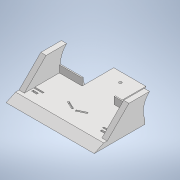
# Autodesk Inventor part: dół
Saved by Autodesk Inventor 2022 (Build 260153000, 153)
## iProperties
Created: 2022-12-08
Part Number: dół
Material: Generic
Document SubType Name: Modeling
Designer: Kamil
Density: 1 g/cm^3
Appearance: Default
Author: Kamil
Autodesk Inventor part; units mm, degrees
ref_plane "YZ Plane" through (0, 0, 0) normal (1, 0, 0) x (0, 1, 0)
ref_plane "XZ Plane" through (0, 0, 0) normal (0, 1, 0) x (-1, 0, 0)
ref_plane "XY Plane" through (0, 0, 0) normal (0, 0, 1) x (1, 0, 0)
sketch "Sketch1" plane through (0, 0, 0) normal (0, 1, 0) x (-1, 0, 0)
  line L0 (-49.6221, -50.9693) -> (50.3779, -50.9693)
  line L1 (50.3779, -50.9693) -> (50.3779, 49.0307)
  line L2 (50.3779, 49.0307) -> (-49.6221, 49.0307)
  line L3 (-49.6221, 49.0307) -> (-49.6221, -50.9693)
  line L4 (-17.8721, -0.5117) -> (18.6279, -0.5117)
  line L5 (18.6279, -0.5117) -> (18.6279, -50.9693)
  line L6 (18.6279, -50.9693) -> (-17.8721, -50.9693)
  line L7 (-17.8721, -50.9693) -> (-17.8721, -0.5117)
  line L8 (-49.6221, -18.7693) -> (50.3779, -18.7693)
  line L9 (50.3779, -18.7693) -> (50.3779, -50.9693)
  line L10 (50.3779, -50.9693) -> (-49.6221, -50.9693)
  line L11 (-49.6221, -50.9693) -> (-49.6221, -18.7693)
  line L12 (-49.6221, -18.7693) -> (50.3779, -18.7693)
  line L13 (50.3779, -18.7693) -> (50.3779, -14.7693)
  line L14 (50.3779, -14.7693) -> (-49.6221, -14.7693)
  line L15 (-49.6221, -14.7693) -> (-49.6221, -18.7693)
  line L16 (-49.6221, -34.8693) -> (50.3779, -34.8693)
  line L17 (-49.6221, -50.9693) -> (50.3779, -50.9693)
  line L18 (50.3779, -50.9693) -> (50.3779, -46.9693)
  line L19 (50.3779, -46.9693) -> (-49.6221, -46.9693)
  line L20 (-49.6221, -46.9693) -> (-49.6221, -50.9693)
  point P0 (0, 0)
  point P1 (0.3779, -50.9693)
  point P2 (0.3779, -50.9693)
  point P3 (0.3779, -50.9693)
  point P4 (-49.6221, -14.7693)
  point P5 (-17.8721, -14.7693)
  point P6 (-17.8721, -46.9693)
  point P7 (18.6279, -46.9693)
  point P8 (18.6279, -14.7693)
  dimension "d0" = 100
  dimension "d1" = 100
  dimension "d2" = 36.5
  dimension "d3" = 100
  dimension "d4" = 32.2
  dimension "d5" = 4
  dimension "d6" = 4
  constraints: 42 end point, 10 parallel, 5 horizontal, 5 midpoint, 5 perpendicular, 2 point on line
  measures "d0" distance of L2.end L1.end
  measures "d1" distance of L1.end L0.end
  measures "d2" distance of L5.end L6.end
  measures "d3" distance of L9.end L10.end
  measures "d4" distance of L8.end L9.end
  measures "d5" distance of L13.end L12.end
  measures "d6" distance of L18.end L17.end
extrude "Extrusion1" add sketch "Sketch1" along normal blind 4 contours L7 L16 L5 L19 | L7 L8 L5 L16 | L7 L14 L5 L8 | L3 L2 L1 L14 L5 L4 L7 | L7 L4 L5 L14
sketch "Sketch2" plane through (17.8721, 0, -14.7693) normal (1, 0, 0) x (0, 0, -1)
  line L0 (0, 0) -> (32.2, 0) projected
  line L1 (32.2, 0) -> (32.2, 4) projected
  line L2 (0, 4) -> (32.2, 4) projected
  line L3 (0, 0) -> (0, 4) projected
  circle A0 centre (20.1, 13.6) radius 16.1 projected
  line L4 (32.2, 0) -> (32.2, 4) projected
  circle A1 centre (20.1, 13.6) radius 15.4457
  point P0 (-14.7693, 0)
  point P1 (27.4219, 0)
  constraints: 1 coincident, 3 other
extrude "Extrusion2" cut sketch "Sketch2" against normal through all contours A0 L1 L0 | L0 A1 L1 A0
sketch "Sketch3" plane through (0, 0, 0) normal (0, -1, 0) x (1, 0, 0)
  line L0 (-18.6279, -46.9693) -> (-18.6279, -42.1911) projected
  line L1 (17.8721, -46.9693) -> (-18.6279, -46.9693) projected
  line L2 (17.8721, -42.1911) -> (17.8721, -46.9693) projected
  line L3 (-18.6279, -42.1911) -> (17.8721, -42.1911) projected
  line L4 (-18.6279, -42.1911) -> (17.8721, -42.1911) projected
  line L5 (17.8721, -14.7693) -> (17.8721, -42.1911) projected
  line L6 (49.6221, -14.7693) -> (17.8721, -14.7693) projected
  line L7 (49.6221, 49.0307) -> (49.6221, -14.7693) projected
  line L8 (-50.3779, 49.0307) -> (49.6221, 49.0307) projected
  line L9 (-50.3779, -14.7693) -> (-50.3779, 49.0307) projected
  line L10 (-18.6279, -14.7693) -> (-50.3779, -14.7693) projected
  line L11 (-18.6279, -42.1911) -> (-18.6279, -14.7693) projected
  line L12 (17.8721, -46.9693) -> (-18.6279, -46.9693) projected
  line L13 (-18.6279, -42.1911) -> (17.8721, -42.1911) projected
  line L14 (2.6221, -34.1911) -> (-3.3779, -34.1911)
  line L15 (-3.3779, -34.1911) -> (-3.3779, -42.1911)
  line L16 (-3.3779, -42.1911) -> (2.6221, -42.1911)
  line L17 (2.6221, -42.1911) -> (2.6221, -34.1911)
  line L18 (2.6221, -42.1911) -> (-3.3779, -42.1911)
  line L19 (-3.3779, -42.1911) -> (-3.3779, -53.2472)
  line L20 (-3.3779, -53.2472) -> (2.6221, -53.2472)
  line L21 (2.6221, -53.2472) -> (2.6221, -42.1911)
  point P0 (0, 0)
  point P1 (-0.3779, -46.9693)
  point P2 (-0.3779, -42.1911)
  point P3 (-0.3779, -42.1911)
  dimension "d11" = 6
  dimension "d12" = 8
  constraints: 16 end point, 4 parallel, 3 midpoint, 2 horizontal, 2 perpendicular
  measures "d11" distance of L16.end L15.end
  measures "d12" distance of L15.end L14.end
extrude "Extrusion3" cut sketch "Sketch3" against normal blind 2 contours L19 L3 L21 L1 | L1 L21 L20 L19 | L15 L14 L17 L3
sketch "Sketch4" plane through (0, 4, 0) normal (0, 1, 0) x (1, 0, 0)
  line L0 (49.6221, -49.0307) -> (49.6221, 14.7693) projected
  line L1 (49.6221, 14.7693) -> (17.8721, 14.7693) projected
  line L2 (17.8721, 14.7693) -> (17.8721, 46.9693) projected
  line L3 (17.8721, 46.9693) -> (-18.6279, 46.9693) projected
  line L4 (-18.6279, 46.9693) -> (-18.6279, 14.7693) projected
  line L5 (-18.6279, 14.7693) -> (-50.3779, 14.7693) projected
  line L6 (-50.3779, 14.7693) -> (-50.3779, -49.0307) projected
  line L7 (-50.3779, -49.0307) -> (49.6221, -49.0307) projected
  point P0 (0, 0)
extrude "Extrusion4" add sketch "Sketch4" along normal blind 1
sketch "Sketch5" plane through (17.8721, 0, -14.7693) normal (1, 0, 0) x (0, 0, -1)
  arc A0 (27.4219, 0) -> (32.2, 4) centre (20.1, 13.6) ccw projected
  arc A1 (27.4219, 0) -> (32.2, 4) centre (20.1, 13.6) ccw projected
  circle A2 centre (20.1, 13.6) radius 15.4457
  arc A3 (27.4219, 0) -> (32.2, 4) centre (20.1, 13.6) ccw projected
  line L0 (32.2, 4) -> (32.2, 5) projected
  line L1 (0, 5) -> (32.2, 5) projected
  line L2 (0, 0) -> (0, 5) projected
  line L3 (0, 0) -> (27.4219, 0) projected
  line L4 (32.2, 5) -> (32.93, 5)
  point P0 (-14.7693, 0)
  point P1 (32.2, 4)
  constraints: 2 end point, 2 point on circle, 1 centre point, 1 coincident, 1 horizontal
extrude "Extrusion5" add sketch "Sketch5" against normal up to surface (36.5 mm away) contours L0 L4 A2
sketch "Sketch6" plane through (0, 2, 0) normal (0, -1, 0) x (1, 0, 0)
  line L0 (2.6221, -45.0678) -> (-3.3779, -45.0678) projected
  line L1 (2.6221, -34.1911) -> (2.6221, -45.0678) projected
  line L2 (-3.3779, -34.1911) -> (2.6221, -34.1911) projected
  line L3 (-3.3779, -45.0678) -> (-3.3779, -34.1911) projected
  line L4 (-3.3779, -34.1911) -> (2.6221, -34.1911) projected
  line L5 (-0.3779, -34.1911) -> (-0.3779, -35.8821)
  line L6 (-0.3779, -34.1911) -> (-0.3779, -36.935)
  circle A0 centre (-0.3779, -36.935) radius 1.5
  point P0 (0, 0)
  dimension "d19" = 3
  constraints: 4 end point, 1 centre point, 1 coincident, 1 midpoint, 1 point on line, 1 vertical
  measures "d19" diameter of A0
extrude "Extrusion6" cut sketch "Sketch6" against normal blind 10 contours A0
sketch "Sketch7" plane through (49.6221, 0, 49.0307) normal (1, 0, 0) x (0, 0, -1)
  circle A0 centre (83.9, 13.6) radius 16.1 projected
  line L0 (0, 0) -> (63.8, 0) projected
  line L1 (63.8, 0) -> (63.8, 5) projected
  line L2 (0, 5) -> (63.8, 5) projected
  line L3 (0, 0) -> (0, 5) projected
  arc A1 (91.2219, 0) -> (96.73, 5) centre (83.9, 13.6) ccw projected
  line L4 (63.8, 5) -> (96.73, 5) projected
  line L5 (63.8, 0) -> (63.8, 5) projected
  line L6 (63.8, 0) -> (91.2219, 0) projected
  line L7 (0, 0) -> (63.8, 0) projected
  line L8 (0, 0) -> (0, -14.6713)
  line L9 (83.9, -2.5) -> (-11.8385, -2.5)
  line L10 (91.2219, 0) -> (63.8, 0) projected
  line L11 (3.6899, -2.5) -> (17.1336, 5)
  line L12 (0, 5) -> (63.8, 5) projected
  line L13 (17.1336, 5) -> (28.2336, 16.1)
  line L14 (17.1336, 5) -> (32.8313, 5) construction
  line L15 (28.2336, 16.1) -> (29.6478, 14.6857)
  line L16 (29.6478, 14.6857) -> (19.962, 5)
  line L17 (83.9, 29.7) -> (9.0674, 29.7)
  line L18 (29.6478, 14.6857) -> (44.662, 29.7)
  line L19 (63.8, 5) -> (96.73, 5) projected
  circle A2 centre (83.9, 13.6) radius 21.8625
  line L20 (17.1336, 5) -> (1.0083, -2.5)
  point P0 (49.0307, 0)
  point P1 (6.3834, 0)
  dimension "d22" = 45
  dimension "d23" = 2
  constraints: 20 end point, 5 point on line, 2 horizontal, 2 perpendicular, 2 point on circle, 2 tangent, 1 coincident, 1 equal length, 1 parallel, 1 vertical, 3 other
  measures "d22" angle of L14 L13
  measures "d23" distance of L13.end L15.end
extrude "Extrusion7" cut sketch "Sketch7" against normal through all contours L20 L0 L3 L2
sketch "Sketch8" plane through (49.6221, 0, -14.7693) normal (1, 0, 0) x (0, 0, -1)
  line L0 (-46.6664, 5) -> (-57.4166, 0) projected
  line L1 (-57.4166, 0) -> (0, 0) projected
  line L2 (0, 0) -> (0, 5) projected
  line L3 (-46.6664, 5) -> (0, 5) projected
  line L4 (0, 5) -> (-46.6664, 5) projected
  line L5 (-45.5728, 5) -> (-39.1497, 11.4231)
  line L6 (-45.5728, 5) -> (-36.4892, 5) construction
  line L7 (-39.1497, 11.4231) -> (-37.7355, 10.0089)
  line L8 (-37.7355, 10.0089) -> (-42.7444, 5)
  line L9 (-42.7444, 5) -> (-5.7272, 42.0172)
  circle A0 centre (20.1, 13.6) radius 16.1 projected
  line L10 (20.1, 29.7) -> (-35.8827, 29.7)
  line L11 (32.93, 5) -> (0, 5) projected
  circle A1 centre (20.1, 13.6) radius 21.8625
  point P0 (-14.7693, 0)
  point P1 (5.3095, 29.7)
  point P2 (-18.0444, 29.7)
  dimension "d26" = 45
  dimension "d27" = 2
  constraints: 12 end point, 3 horizontal, 2 point on line, 1 coincident, 1 equal length, 1 perpendicular, 1 vertical alignment, 4 other
  measures "d26" angle of L6 L5
  measures "d27" distance of L5.end L7.end
extrude "Extrusion8" add sketch "Sketch8" against normal blind 6 contours L8 L9 L10 A1 L3
sketch "Sketch9" plane through (-50.3779, 0, -14.7693) normal (-1, 0, 0) x (0, 0, 1)
  line L0 (57.4166, 0) -> (46.6664, 5) projected
  line L1 (0, 5) -> (46.6664, 5) projected
  line L2 (0, 0) -> (0, 5) projected
  line L3 (0, 0) -> (57.4166, 0) projected
  line L4 (18.0444, 29.7) -> (-5.3095, 29.7) projected
  arc A0 (0, 5) -> (-5.3095, 29.7) centre (-20.1, 13.6) ccw projected
  line L5 (42.7444, 5) -> (0, 5) projected
  line L6 (42.7444, 5) -> (18.0444, 29.7) projected
  point P0 (14.7693, 0)
extrude "Extrusion9" add sketch "Sketch9" against normal blind 6 contours L1 A0 L4 L6
sketch "Sketch10" plane through (0, 5, 0) normal (0, 1, 0) x (1, 0, 0)
  line L0 (-44.3779, -27.9751) -> (-50.3779, -27.9751) projected
  line L1 (-50.3779, -27.9751) -> (-50.3779, -31.8971) projected
  line L2 (-50.3779, -31.8971) -> (49.6221, -31.8971) projected
  line L3 (49.6221, -31.8971) -> (49.6221, -27.9751) projected
  line L4 (49.6221, -27.9751) -> (43.6221, -27.9751) projected
  line L5 (43.6221, -27.9751) -> (43.6221, 14.7693) projected
  line L6 (43.6221, 14.7693) -> (17.8721, 14.7693) projected
  line L7 (17.8721, 14.7693) -> (17.8721, 47.6993) projected
  line L8 (17.8721, 47.6993) -> (-18.6279, 47.6993) projected
  line L9 (-18.6279, 47.6993) -> (-18.6279, 14.7693) projected
  line L10 (-18.6279, 14.7693) -> (-44.3779, 14.7693) projected
  line L11 (-44.3779, 14.7693) -> (-44.3779, -27.9751) projected
  circle A0 centre (-0.3779, 36.935) radius 1.5 projected
  line L12 (43.6221, -27.9751) -> (43.6221, 14.7693) projected
  line L13 (17.8721, 14.7693) -> (43.6221, 14.7693)
  line L14 (43.6221, 14.7693) -> (43.6221, 11.7693)
  line L15 (43.6221, 11.7693) -> (17.8721, 11.7693)
  line L16 (17.8721, 11.7693) -> (17.8721, 14.7693)
  line L17 (-44.3779, 14.7693) -> (-44.3779, -27.9751) projected
  line L18 (-18.6279, 14.7693) -> (-44.3779, 14.7693)
  line L19 (-44.3779, 14.7693) -> (-44.3779, 11.7693)
  line L20 (-44.3779, 11.7693) -> (-18.6279, 11.7693)
  line L21 (-18.6279, 11.7693) -> (-18.6279, 14.7693)
  point P0 (0, 0)
  dimension "d32" = 3
  dimension "d33" = 3
  constraints: 16 end point, 4 parallel, 2 horizontal, 2 perpendicular, 2 point on line
  measures "d32" distance of L13.end L14.end
  measures "d33" distance of L19.end L18.end
extrude "Extrusion10" add sketch "Sketch10" along normal blind 8 contours L11 L10 L21 L20 | L15 L16 L6 L5
sketch "Sketch11" plane through (-50.3779, 0, -14.7693) normal (-1, 0, 0) x (0, 0, 1)
  arc A0 (0, 5) -> (1.7543, 13) centre (-20.1, 13.6) ccw projected
  line L0 (0, 13) -> (1.7543, 13) projected
  line L1 (0, 5) -> (0, 13) projected
  point P0 (14.7693, 0)
extrude "Extrusion11" cut sketch "Sketch11" against normal through all
sketch "Sketch12" plane through (0, 0, 0) normal (0, -1, 0) x (1, 0, 0)
  line L0 (49.6221, 42.6473) -> (-50.3779, 42.6473) projected
  line L1 (-50.3779, -14.7693) -> (-50.3779, 42.6473) projected
  line L2 (-18.6279, -14.7693) -> (-50.3779, -14.7693) projected
  line L3 (-18.6279, -42.1911) -> (-18.6279, -14.7693) projected
  line L4 (-18.6279, -42.1911) -> (-3.3779, -42.1911) projected
  line L5 (-3.3779, -42.1911) -> (-3.3779, -34.1911) projected
  line L6 (-3.3779, -34.1911) -> (2.6221, -34.1911) projected
  line L7 (2.6221, -34.1911) -> (2.6221, -42.1911) projected
  line L8 (2.6221, -42.1911) -> (17.8721, -42.1911) projected
  line L9 (17.8721, -14.7693) -> (17.8721, -42.1911) projected
  line L10 (49.6221, -14.7693) -> (17.8721, -14.7693) projected
  line L11 (49.6221, 42.6473) -> (49.6221, -14.7693) projected
  circle A0 centre (-0.3779, -36.935) radius 1.5 projected
  line L12 (17.8721, -14.7693) -> (17.8721, -47.6993) projected
  line L13 (17.8721, -47.6993) -> (-18.6279, -47.6993) projected
  line L14 (-18.6279, -47.6993) -> (-18.6279, -14.7693) projected
  line L15 (-18.6279, -14.7693) -> (-18.6279, -11.7693) projected
  line L16 (-18.6279, -11.7693) -> (-44.3779, -11.7693) projected
  line L17 (-44.3779, -11.7693) -> (-44.3779, 27.9751) projected
  line L18 (-44.3779, 27.9751) -> (-50.3779, 27.9751) projected
  line L19 (-50.3779, 27.9751) -> (-50.3779, 31.8971) projected
  line L20 (-50.3779, 31.8971) -> (49.6221, 31.8971) projected
  line L21 (49.6221, 31.8971) -> (49.6221, 27.9751) projected
  line L22 (49.6221, 27.9751) -> (43.6221, 27.9751) projected
  line L23 (43.6221, 27.9751) -> (43.6221, -11.7693) projected
  line L24 (43.6221, -11.7693) -> (17.8721, -11.7693) projected
  line L25 (17.8721, -11.7693) -> (17.8721, -14.7693) projected
  line L26 (-44.3779, -11.7693) -> (-44.3779, 27.9751) projected
  line L27 (-44.3779, 27.9751) -> (-42.3779, 27.9751)
  line L28 (-42.3779, 27.9751) -> (-36.3779, 27.9751)
  line L29 (-36.3779, 27.9751) -> (-36.3779, 19.9751)
  line L30 (-36.3779, 19.9751) -> (-42.3779, 19.9751)
  line L31 (-42.3779, 19.9751) -> (-42.3779, 27.9751)
  line L32 (43.6221, 27.9751) -> (43.6221, -11.7693) projected
  line L33 (43.6221, 27.9751) -> (41.6221, 27.9751)
  line L34 (41.6221, 27.9751) -> (35.6221, 27.9751)
  line L35 (35.6221, 27.9751) -> (35.6221, 19.9751)
  line L36 (35.6221, 19.9751) -> (41.6221, 19.9751)
  line L37 (41.6221, 19.9751) -> (41.6221, 27.9751)
  point P0 (0, 0)
  dimension "d38" = 2
  dimension "d39" = 6
  dimension "d40" = 8
  dimension "d41" = 2
  dimension "d42" = 6
  constraints: 20 end point, 4 horizontal, 4 parallel, 2 perpendicular
  measures "d38" distance of L17.end L27.end
  measures "d39" distance of L29.end L30.end
  measures "d40" distance of L28.end L29.end
  measures "d41" distance of L22.end L33.end
  measures "d42" distance of L36.end L35.end
extrude "Extrusion12" cut sketch "Sketch12" against normal blind 2 contours L28 L29 L30 L31 | L37 L36 L35 L34
sketch "Sketch13" plane through (0, 2, 0) normal (0, -1, 0) x (1, 0, 0)
  line L0 (35.6221, 19.9751) -> (35.6221, 27.9751) projected
  line L1 (41.6221, 19.9751) -> (35.6221, 19.9751) projected
  line L2 (41.6221, 27.9751) -> (41.6221, 19.9751) projected
  line L3 (35.6221, 27.9751) -> (41.6221, 27.9751) projected
  line L4 (-36.3779, 19.9751) -> (-42.3779, 19.9751) projected
  line L5 (-36.3779, 27.9751) -> (-36.3779, 19.9751) projected
  line L6 (-42.3779, 27.9751) -> (-36.3779, 27.9751) projected
  line L7 (-42.3779, 19.9751) -> (-42.3779, 27.9751) projected
  line L8 (-36.3779, 27.9751) -> (-36.3779, 19.9751) projected
  line L9 (-42.3779, 19.9751) -> (-36.3779, 19.9751)
  line L10 (-36.3779, 19.9751) -> (-36.3779, 21.9751)
  line L11 (-36.3779, 21.9751) -> (-42.3779, 21.9751)
  line L12 (-42.3779, 21.9751) -> (-42.3779, 19.9751)
  line L13 (41.6221, 27.9751) -> (41.6221, 19.9751) projected
  line L14 (35.6221, 19.9751) -> (35.6221, 27.9751) projected
  line L15 (41.6221, 19.9751) -> (35.6221, 19.9751)
  line L16 (35.6221, 19.9751) -> (35.6221, 21.9751)
  line L17 (35.6221, 21.9751) -> (41.6221, 21.9751)
  line L18 (41.6221, 21.9751) -> (41.6221, 19.9751)
  point P0 (0, 0)
  dimension "d45" = 2
  constraints: 16 end point, 4 parallel, 3 point on line, 2 horizontal, 2 perpendicular
  measures "d45" distance of L10.end L9.end
extrude "Extrusion13" cut sketch "Sketch13" against normal through all contours L0 L17 L2 L1 | L4 L7 L11 L5
body "Solid1"
